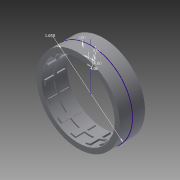
# Autodesk Inventor part: TireDE
Saved by Autodesk Inventor 2015 (Build 190159000, 159)
## iProperties
Created: 2017-12-12
Part Number: TireDE
Material: Generic
Document SubType Name: Modeling
Designer: Administrator
Density: 1 g/cm^3
Appearance: Default
Author: Administrator
Autodesk Inventor part; units mm, degrees
ref_plane "YZ Plane" through (0, 0, 0) normal (1, 0, 0) x (0, 1, 0)
ref_plane "XZ Plane" through (0, 0, 0) normal (0, 1, 0) x (-1, 0, 0)
ref_plane "XY Plane" through (0, 0, 0) normal (0, 0, 1) x (1, 0, 0)
sketch "Sketch1" plane through (0, 0, 0) normal (0, 0, 1) x (1, 0, 0)
  circle A0 centre (0, 0) radius 20.955
  circle A1 centre (0, 0) radius 18.415
  arc A2 (1.2314, 17.61) -> (-1.2314, 17.61) centre (0, 0) ccw
  line L0 (0, 0) -> (0, 23.4982) construction
  line L1 (1.2314, 17.61) -> (1.2846, 18.3701)
  line L2 (-1.2314, 17.61) -> (-1.2846, 18.3701)
  dimension "d0" = 41.91
  dimension "d1" = 2.54
  dimension "d2" = 0.762
  dimension "d3" = 4
  dimension "d5" = 4
  constraints: 6 end point, 4 point on circle, 3 centre point, 3 coincident, 1 vertical
  measures "d0" diameter of A0
  measures "d1" radial gap between concentric circles of A0 A1
  measures "d2" radial gap between concentric circles of A1 A2
  measures "d3" angle of L0 L1
  measures "d5" angle of L0 L2
extrude "Extrusion1" add sketch "Sketch1" along normal mid plane 12.7
extrude "Extrusion2" add sketch "Sketch1" along normal mid plane 10.16 contours L1 A2 L2 A1 picked at (-0.1369, 18.1561)
pattern_circular "Circular Pattern1" count 15 over 360 about axis through (0, 0, 0) along (0, 0, 1) of "Extrusion2"
ref_plane "Work Plane1" through (0, 0, 0) normal (0, 0, 1) x (1, 0, 0)
sketch "Sketch2" plane through (0, 0, 0) normal (0, 0, 1) x (1, 0, 0)
  circle A0 centre (0, 0) radius 19.3779
  circle A1 centre (0, 0) radius 17.653
  constraints: 2 centre point, 2 coincident
extrude "Extrusion3" add sketch "Sketch2" along normal mid plane 1.27
body "Solid1"
